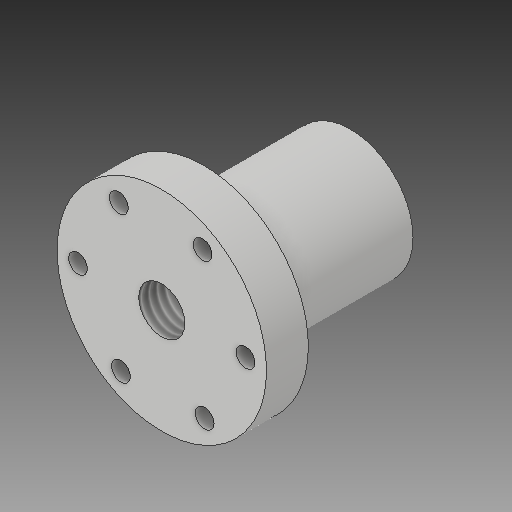
# Autodesk Inventor part: nut
Saved by Autodesk Inventor 2018 (Build 220112000, 112)
## iProperties
Created: 2017-06-20
Part Number: nut
Material: Generic
Document SubType Name: Modeling
Designer: M228544
Density: 1 g/cm^3
Appearance: Default
Author: M228544
Autodesk Inventor part; units mm, degrees
ref_plane "YZ Plane" through (0, 0, 0) normal (1, 0, 0) x (0, 1, 0)
ref_plane "XZ Plane" through (0, 0, 0) normal (0, 1, 0) x (-1, 0, 0)
ref_plane "XY Plane" through (0, 0, 0) normal (0, 0, 1) x (1, 0, 0)
sketch "Sketch1" plane through (0, 0, 0) normal (0, 1, 0) x (-1, 0, 0)
  line L0 (0, 0) -> (-25, 0)
  line L1 (-25, 0) -> (-25, -10)
  line L2 (-25, -10) -> (-15, -10)
  line L3 (-15, -10) -> (-15, -45)
  line L4 (-15, -45) -> (0, -45)
  line L5 (0, 0) -> (0, -45)
  dimension "d3" = 25
  dimension "d4" = 10
  dimension "d5" = 10
  dimension "d6" = 35
  dimension "d7" = 15
  constraints: 12 end point, 4 perpendicular, 1 horizontal
  measures "d3" distance of L0.start L0.end
  measures "d4" distance of L0.end L1.end
  measures "d5" distance of L1.end L2.end
  measures "d6" distance of L2.end L3.end
  measures "d7" distance of L3.end L4.end
revolve "Revolution1" add sketch "Sketch1" angle 360 about axis through (0, 0, 0) along (0, 0, -1)
sketch "Sketch2" plane through (0, 0, 0) normal (0, 0, 1) x (1, 0, 0)
  line L0 (0, 0) -> (30.242, 0) construction
  line L1 (0, 0.5707) -> (22.435, 0.5707) construction
  circle A0 centre (9.7519, 17.4614) radius 2.25
  circle A1 centre (19.998, 0.2854) radius 2.25
  circle A2 centre (10.2461, -17.1761) radius 2.25
  circle A3 centre (-9.7519, -17.4614) radius 2.25
  circle A4 centre (-19.998, -0.2854) radius 2.25
  circle A5 centre (-10.2461, 17.1761) radius 2.25
  dimension "d12" = 4.5
  dimension "d15" = 360
  constraints: 6 centre point, 4 end point, 2 horizontal, 1 coincident, 13 other
  measures "d12" diameter of A0
extrude "Extrusion1" cut sketch "Sketch2" against normal through all
sketch "Sketch3" plane through (0, 0, 0) normal (0, 0, 1) x (1, 0, 0)
  circle A0 centre (0, 0) radius 5.5
  dimension "d19" = 11
  constraints: 1 centre point, 1 coincident
  measures "d19" diameter of A0
extrude "Extrusion2" cut sketch "Sketch3" against normal through all
thread "Thread1" size "1/2-13 UNC" class "2B" standard "ANSI Unified Screw Threads" full length
body "Solid1"
